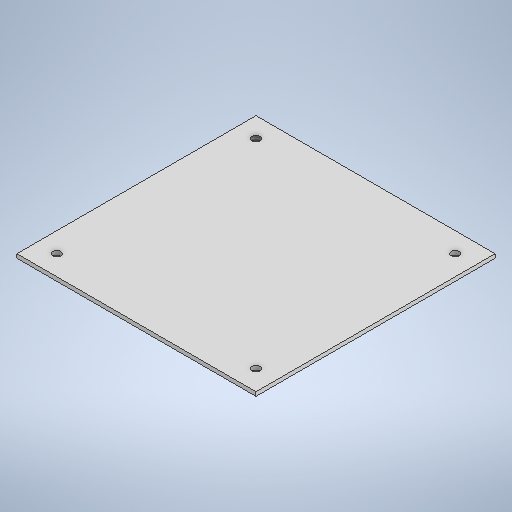
# Autodesk Inventor part: PCB
Saved by Autodesk Inventor 2025 (Build 290162000, 162)
## iProperties
Created: 2024-04-10
Part Number: PCB
Material: Generic
Document SubType Name: Modeling
Designer: mahal
Density: 1 g/cm^3
Appearance: Default
Author: mahal
Autodesk Inventor part; units mm, degrees
ref_plane "YZ Plane" through (0, 0, 0) normal (1, 0, 0) x (0, 1, 0)
ref_plane "XZ Plane" through (0, 0, 0) normal (0, 1, 0) x (-1, 0, 0)
sketch "Sketch1" plane through (0, 0, 0) normal (0, 1, 0) x (-1, 0, 0)
  line L0 (60, 60) -> (-60, 60)
  line L1 (-60, 60) -> (-60, -60)
  line L2 (-60, -60) -> (60, -60)
  line L3 (60, -60) -> (60, 60)
  line L4 (60, 60) -> (-60, -60) construction
  line L5 (-60, 60) -> (60, -60) construction
  point P0 (0, 0)
  dimension "d0" = 120
  dimension "d1" = 120
  constraints: 12 end point, 2 midpoint, 2 parallel, 1 horizontal, 1 perpendicular
  measures "d0" distance of L2.end L1.end
  measures "d1" distance of L1.end L0.end
extrude "Extrusion1" add sketch "Sketch1" along normal blind 2
ref_plane "Work Plane1" through (0, 2, 0) normal (0, 1, 0) x (1, 0, 0)
sketch "Sketch2" plane through (0, 2, 0) normal (0, 1, 0) x (1, 0, 0)
  line L0 (60, 60) -> (-60, 60) projected
  line L1 (59.4693, -59.8704) -> (-60, 60)
  circle A0 centre (-50, 50) radius 2
  line L2 (0, 60) -> (0, 51.4464)
  circle A1 centre (50, 50) radius 2
  line L3 (60, -60) -> (60, 60) projected
  line L4 (60, 0) -> (52.6499, 0)
  circle A2 centre (50, -50) radius 2
  line L5 (-60, 60) -> (-60, -60) projected
  line L6 (-60, 0) -> (-53.051, 0)
  circle A3 centre (-50, -50) radius 2
  point P0 (0, 0)
  dimension "d5" = 4
  constraints: 8 end point, 4 centre point, 3 midpoint, 3 symmetric about line, 2 horizontal, 1 vertical, 3 other
  measures "d5" diameter of A0
extrude "Extrusion2" cut sketch "Sketch2" against normal through all
thread "Thread1" size "M9x1.25" class "6H" standard "ANSI Metric M Profile" full length
body "Solid1"
